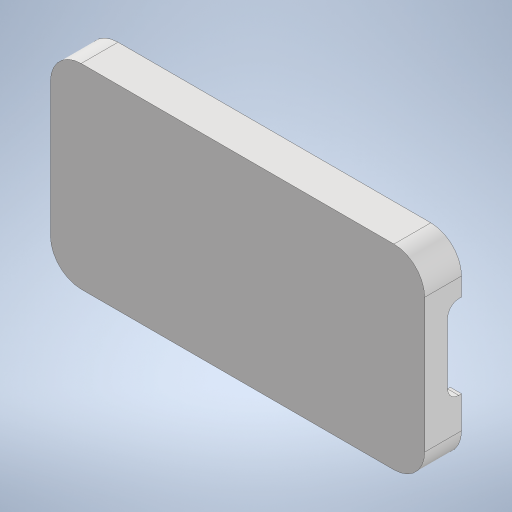
# Autodesk Inventor part: case_base
Saved by Autodesk Inventor 2023 (Build 270158000, 158)
## iProperties
Created: 2024-10-24
Part Number: case_base
Material: Generic
Document SubType Name: Modeling
Designer: lwerne
Density: 1 g/cm^3
Appearance: Default
Author: lwerne
Autodesk Inventor part; units mm, degrees
ref_plane "YZ Plane" through (0, 0, 0) normal (1, 0, 0) x (0, 1, 0)
ref_plane "XZ Plane" through (0, 0, 0) normal (0, 1, 0) x (-1, 0, 0)
sketch "Sketch1" plane through (0, 0, 0) normal (0, 0, 1) x (1, 0, 0)
  circle A0 centre (28, -12) radius 1.6 construction
  circle A1 centre (-25, -0.5) radius 1.6 construction
  circle A2 centre (28, 12) radius 1.6 construction
  line L0 (-28, -15) -> (28, -15)
  line L1 (-31, 12) -> (-31, -12)
  line L2 (28, 15) -> (-28, 15)
  line L3 (31, -12) -> (31, 12)
  circle A3 centre (28, -12) radius 3
  circle A4 centre (28, 12) radius 3
  circle A5 centre (-25, -0.5) radius 3
  circle A6 centre (28, -12) radius 1.4
  circle A7 centre (28, 12) radius 1.4
  circle A8 centre (-25, -0.5) radius 1.4
  point P0 (0, 0)
extrude "Extrusion1" add sketch "Sketch1" along normal blind 3
sketch "Sketch2" plane through (28, -12, 3) normal (0, 0, 1) x (1, 0, 0)
  line L0 (-59, 24) -> (-59, 0) projected
  line L1 (0, 27) -> (-56, 27) projected
  line L2 (-56, -3) -> (0, -3) projected
  line L3 (3, 0) -> (3, 24) projected
  line L4 (-59, 27) -> (3, 27)
  line L5 (3, 27) -> (3, -3)
  line L6 (3, -3) -> (-59, -3)
  line L7 (-59, -3) -> (-59, 27)
  point P0 (-28, 12)
  constraints: 8 end point, 2 parallel, 1 horizontal, 1 perpendicular
extrude "Extrusion2" add sketch "Sketch2" along normal blind 2
fillet "Fillet1" radius 3 4 edges at (31, -15, 4) (31, 15, 4) (-31, 15, 4) (-31, -15, 4)
sketch "Sketch3" plane through (28, -12, 5) normal (0, 0, 1) x (1, 0, 0)
  arc A0 (-59, 0) -> (-56, -3) centre (-56, 0) ccw projected
  line L0 (-56, -3) -> (0, -3) projected
  arc A1 (0, -3) -> (3, 0) centre (0, 0) ccw projected
  line L1 (3, 0) -> (3, 24) projected
  arc A2 (3, 24) -> (0, 27) centre (0, 24) ccw projected
  line L2 (0, 27) -> (-56, 27) projected
  arc A3 (-56, 27) -> (-59, 24) centre (-56, 24) ccw projected
  line L3 (-59, 24) -> (-59, 0) projected
  line L4 (5.5, 24) -> (5.5, 0)
  arc A4 (0, -5.5) -> (5.5, 0) centre (0, 0) ccw
  line L5 (0, -5.5) -> (-56, -5.5)
  arc A5 (-61.5, 0) -> (-56, -5.5) centre (-56, 0) ccw
  line L6 (-61.5, 0) -> (-61.5, 24)
  arc A6 (-56, 29.5) -> (-61.5, 24) centre (-56, 24) ccw
  line L7 (-56, 29.5) -> (0, 29.5)
  arc A7 (5.5, 24) -> (0, 29.5) centre (0, 24) ccw
  point P0 (-28, 12)
  dimension "d9" = 2.5
  constraints: 8 end point, 8 point on circle, 4 centre point, 7 other
  measures "d9" distance between parallel lines of L1 L4
ref_plane "Work Plane1" through (-31, -15, -1.6) normal (0, 0, -1) x (0, 1, 0)
extrude "Extrusion3" add sketch "Sketch3" against normal up to surface (6.6 mm away)
sketch "Sketch4" plane through (28, 17.5, -1.6) normal (0, 0, -1) x (-1, 0, 0)
  arc A0 (59, -5.5) -> (56, -2.5) centre (56, -5.5) ccw projected
  line L0 (59, -29.5) -> (59, -5.5) projected
  arc A1 (56, -32.5) -> (59, -29.5) centre (56, -29.5) ccw projected
  line L1 (0, -32.5) -> (56, -32.5) projected
  arc A2 (-3, -29.5) -> (0, -32.5) centre (0, -29.5) ccw projected
  line L2 (-3, -5.5) -> (-3, -29.5) projected
  arc A3 (0, -2.5) -> (-3, -5.5) centre (0, -5.5) ccw projected
  line L3 (56, -2.5) -> (0, -2.5) projected
  arc A4 (56, -35) -> (61.5, -29.5) centre (56, -29.5) ccw projected
  line L4 (61.5, -5.5) -> (61.5, -29.5) projected
  arc A5 (61.5, -5.5) -> (56, 0) centre (56, -5.5) ccw projected
  line L5 (0, 0) -> (56, 0) projected
  arc A6 (0, 0) -> (-5.5, -5.5) centre (0, -5.5) ccw projected
  line L6 (-5.5, -29.5) -> (-5.5, -5.5) projected
  arc A7 (-5.5, -29.5) -> (0, -35) centre (0, -29.5) ccw projected
  line L7 (56, -35) -> (0, -35) projected
  arc A8 (0, -2) -> (-3.5, -5.5) centre (0, -5.5) ccw
  line L8 (-3.5, -5.5) -> (-3.5, -29.5)
  arc A9 (-3.5, -29.5) -> (0, -33) centre (0, -29.5) ccw
  line L9 (0, -33) -> (56, -33)
  arc A10 (56, -33) -> (59.5, -29.5) centre (56, -29.5) ccw
  line L10 (59.5, -29.5) -> (59.5, -5.5)
  arc A11 (59.5, -5.5) -> (56, -2) centre (56, -5.5) ccw
  line L11 (56, -2) -> (0, -2)
  point P0 (28, -17.5)
  dimension "d12" = 0.5
  constraints: 8 end point, 8 point on circle, 4 centre point, 7 other
  measures "d12" distance between parallel lines of L3 L11
extrude "Extrusion4" cut sketch "Sketch4" against normal up to surface (1.6 mm away) contours L11 A11 L10 A10 L9 A9 L8 A8
sketch "Sketch5" plane through (33.5, -12, 5) normal (1, 0, 0) x (0, 0, -1)
  line L0 (6.6, 20.7422) -> (10.115, 20.7422) projected
  line L1 (10.115, 5.7422) -> (6.6, 5.7422) projected
  line L2 (6.6, 20.7422) -> (4.1, 20.7422)
  line L3 (4.1, 20.7422) -> (4.1, 5.7422)
  line L4 (4.1, 5.7422) -> (6.6, 5.7422)
  line L5 (6.6, 5.7422) -> (6.6, 20.7422)
  point P0 (5, 12)
  dimension "d15" = 2.5
  constraints: 8 end point, 2 parallel, 1 horizontal, 1 perpendicular
  measures "d15" distance of L4.end L3.end
extrude "Extrusion5" cut sketch "Sketch5" against normal blind 21.75
fillet "Fillet2" radius 2 2 edges at (32.25, 8.7422, 0.9) (32.25, -6.2578, 0.9)
fillet "Fillet3" radius 2 4 edges at (31, 12, 1.5) (28, 15, 1.5) (28, -15, 1.5) (31, -12, 1.5)
fillet "Fillet4" radius 2 1 edges at (-28, -0.5, 3)
body "Solid1"
